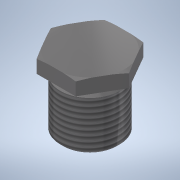
# Autodesk Inventor part: Korek sześciokątny BSP 1/2'' L=25
Saved by Autodesk Inventor 2020 (Build 240168000, 168)
## iProperties
RuleStatus: InUse
Created: 2022-03-21
Part Number: Korek sześciokątny BSP 1/2'' L=25
Material: 304
Description: Korek sześciokątny BSP 1/2'' L=25
Document SubType Name: Modelowanie
Designer: Radosław
Density: 8 g/cm^3
Sheet Metal Rule: 1,5
Sheet Metal Width: 0,000 mm
Sheet Metal Length: 0,000 mm
Sheet Metal Area: 0,000 mm^2
Appearance: Częściowo polerowany(1)
Author: Radosław
Autodesk Inventor part; units mm, degrees
ref_plane "YZ Plane" through (0, 0, 0) normal (1, 0, 0) x (0, 1, 0)
ref_plane "XZ Plane" through (0, 0, 0) normal (0, 1, 0) x (-1, 0, 0)
ref_plane "XY Plane" through (0, 0, 0) normal (0, 0, 1) x (1, 0, 0)
sketch "Szkic7" plane through (0, 0, 0) normal (0, 0, 1) x (1, 0, 0)
  circle A0 centre (0, 0) radius 10.4775
  dimension "d35" = 20.955
  constraints: 1 centre point, 1 coincident
  measures "d35" diameter of A0
extrude "Wyciągnięcie proste2" add sketch "Szkic7" along normal mid plane 18.4375
chamfer "Faza2" distance 1 angle 45 1 edges at (-10.4775, 0, 9.2188)
sketch "Szkic9" plane through (0, 0, 9.2188) normal (0, 0, 1) x (1, 0, 0)
  circle A0 centre (0, 0) radius 9.4775 projected
extrude "Wyciągnięcie proste3" add sketch "Szkic9" along normal blind 1.5625
sketch "Szkic10" plane through (0, 0, 10.7812) normal (0, 0, 1) x (1, 0, 0)
  line L0 (-6.9282, 12) -> (6.9282, 12)
  line L1 (6.9282, 12) -> (13.8564, 0)
  line L2 (13.8564, 0) -> (6.9282, -12)
  line L3 (6.9282, -12) -> (-6.9282, -12)
  line L4 (-6.9282, -12) -> (-13.8564, 0)
  line L5 (-13.8564, 0) -> (-6.9282, 12)
  line L6 (0, 14.6685) -> (0, -14.6685) construction
  line L7 (-14.6685, 0) -> (14.6685, 0) construction
  point P0 (0, 0)
  point P1 (0, 0)
  point P2 (0, 12)
  dimension "d44" = 24
  constraints: 12 end point, 2 point on line, 1 coincident, 1 midpoint, 13 other
  measures "d44" distance between parallel lines of L4 L1
extrude "Wyciągnięcie proste4" add sketch "Szkic10" along normal blind 5
sketch "Szkic12" plane through (0, 0, 0) normal (0, 1, 0) x (-1, 0, 0)
  line L0 (0, -2.1463) -> (0, 12.8775) construction
  line L1 (-6.9282, 10.7812) -> (-6.9282, 15.7812) construction
  line L2 (-13.8564, 15.7812) -> (-6.9282, 15.7812) construction
  line L3 (-13.8564, 10.7812) -> (-13.8564, 15.7812) projected
  line L4 (-13.8564, 15.3525) -> (-12.2564, 15.7812)
  line L5 (-13.8564, 15.7812) -> (-6.9282, 15.7812) projected
  line L6 (-13.8564, 10.7812) -> (-6.9282, 10.7812) projected
  point P0 (0, 0)
  dimension "d50" = 15
  dimension "d51" = 1.6
  constraints: 2 end point, 2 point on line
  measures "d50" angle of L2 L4
  measures "d51" distance from line of L3 L4.end
revolve "Obrót2" cut sketch "Szkic12" angle 360 about axis through (0, 0, -10) along (0, 0, 1)
thread "Gwint3" size "G20.955x1.814" designation "G 1/2" class "A" standard "ISO Pipe Threads" full length
chamfer "Faza3" distance 1 angle 45 1 edges at (-10.4775, 0, -9.2188)
equation "\"d35\" = OD"
equation "\"d36\" = 0.7375 * L"
equation "\"d42\" = 0.0625 * L"
equation "\"d44\" = SW"
equation "\"d45\" = 0.2 * L"
equation "\"d51\" = 0.0666667 * SW"
equation "\"SzerokośćGięciaPodcięcia\" = Grubość"
equation "\"RozmiarPodcięciaNarożnika\" = 4 * Grubość"
equation "\"PromieńPrzejścia\" = PromieńGięcia"
equation "\"Rozmiar_promienia_Jacobiego\" = PromieńGięcia"
equation "\"Wielk_odstępu\" = Grubość"
equation "\"d2\" = PromieńGięcia"
equation "\"d23\" = PromieńGięcia"
equation "\"OD\" = 20.955"
equation "\"SW\" = 24"
equation "\"L\" = 25"
equation "\"Grubość\" = 1.5"
equation "\"PromieńGięcia\" = 3"
